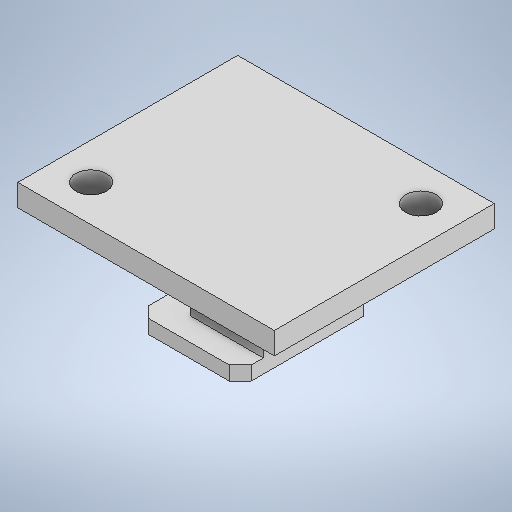
# Autodesk Inventor part: hotshouh mount
Saved by Autodesk Inventor 2025.1 (Build 291241000, 241)
## iProperties
Created: 2025-02-01
Part Number: hotshouh mount
Material: Generisch
Document SubType Name: Modeling
Designer: joebe
Density: 1 g/cm^3
Appearance: Vorgabe
Author: joebe
Autodesk Inventor part; units mm, degrees
ref_plane "YZ Plane" through (0, 0, 0) normal (1, 0, 0) x (0, 1, 0)
ref_plane "XZ Plane" through (0, 0, 0) normal (0, 1, 0) x (-1, 0, 0)
ref_plane "XY Plane" through (0, 0, 0) normal (0, 0, 1) x (1, 0, 0)
sketch "Skizze1" plane through (0, 0, 0) normal (0, 0, 1) x (1, 0, 0)
  line L0 (-7, 9.15) -> (7, 9.15)
  line L1 (7, 9.15) -> (7, -9.15)
  line L2 (7, -9.15) -> (-7, -9.15)
  line L3 (-7, -9.15) -> (-7, 9.15)
  line L4 (-7, 9.15) -> (7, -9.15) construction
  line L5 (7, 9.15) -> (-7, -9.15) construction
  point P0 (0, 0)
  dimension "d0" = 14
  dimension "d1" = 18.3
  constraints: 12 end point, 2 midpoint, 2 parallel, 1 horizontal, 1 perpendicular
  measures "d0" distance of L1.end L2.end
  measures "d1" distance of L0.end L1.end
extrude "Extrusion1" add sketch "Skizze1" along normal blind 1.9
chamfer "Fasen1" distance 1.5 angle 45 4 edges at (-7, -9.15, 0.95) (7, -9.15, 0.95) (7, 9.15, 0.95) (-7, 9.15, 0.95)
sketch "Skizze2" plane through (0, 0, 1.9) normal (0, 0, 1) x (1, 0, 0)
  line L0 (7, -6) -> (-3, -6)
  line L1 (-3, -6) -> (-3, 6)
  line L2 (-3, 6) -> (7, 6)
  line L3 (7, 6) -> (7, -6)
  point P0 (0, 0)
  point P1 (7, 7.65)
  point P2 (-3, 0)
  dimension "d7" = 10
  dimension "d8" = 12
  constraints: 8 end point, 2 parallel, 1 horizontal, 1 horizontal alignment, 1 midpoint, 1 perpendicular, 1 vertical alignment
  measures "d7" distance of L1.end L2.end
  measures "d8" distance of L0.end L1.end
extrude "Extrusion2" add sketch "Skizze2" along normal blind 10
sketch "Skizze3" plane through (0, 0, 11.9) normal (0, 0, 1) x (1, 0, 0)
  line L0 (-17.5, 15) -> (17.5, 15)
  line L1 (17.5, 15) -> (17.5, -15)
  line L2 (17.5, -15) -> (-17.5, -15)
  line L3 (-17.5, -15) -> (-17.5, 15)
  line L4 (-17.5, 15) -> (17.5, -15) construction
  line L5 (17.5, 15) -> (-17.5, -15) construction
  point P0 (0, 0)
  dimension "d11" = 35
  dimension "d12" = 30
  constraints: 12 end point, 2 midpoint, 2 parallel, 1 horizontal, 1 perpendicular
  measures "d11" distance of L1.end L2.end
  measures "d12" distance of L0.end L1.end
extrude "Extrusion3" add sketch "Skizze3" along normal blind 3
sketch "Skizze4" plane through (0, 0, 11.9) normal (0, 0, -1) x (-1, 0, 0)
  line L0 (12.5, -10) -> (-12.5, -10)
  line L1 (-12.5, -10) -> (-12.5, 10)
  line L2 (-12.5, 10) -> (12.5, 10)
  line L3 (12.5, 10) -> (12.5, -10)
  line L4 (12.5, -10) -> (-12.5, 10) construction
  line L5 (-12.5, -10) -> (12.5, 10) construction
  point P0 (0, 0)
  dimension "d15" = 25
  dimension "d16" = 20
  constraints: 12 end point, 2 midpoint, 2 parallel, 1 horizontal, 1 perpendicular
  measures "d15" distance of L1.end L2.end
  measures "d16" distance of L0.end L1.end
hole "Bohrung1" at (-12.5, -10, 11.9) at (12.5, 10, 11.9) direction (0, 0, 1) diameter 4.2 end through all
